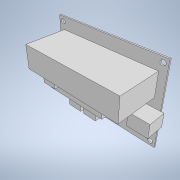
# Autodesk Inventor part: Плата
Saved by Autodesk Inventor 2021.1 (Build 251245010, 245A)
## iProperties
Created: 2026-06-02
Part Number: Плата
Material: Типовые
Document SubType Name: Modeling
Designer: Андрей Тарасов
Density: 1 g/cm^3
Appearance: По умолчанию
Author: Андрей Тарасов
Autodesk Inventor part; units mm, degrees
ref_plane "YZ Plane" through (0, 0, 0) normal (1, 0, 0) x (0, 1, 0)
ref_plane "XZ Plane" through (0, 0, 0) normal (0, 1, 0) x (-1, 0, 0)
ref_plane "XY Plane" through (0, 0, 0) normal (0, 0, 1) x (1, 0, 0)
sketch "Эскиз1" plane through (0, 0, 0) normal (0, 0, 1) x (1, 0, 0)
  line L0 (36.5, -27) -> (-36.5, -27)
  line L1 (-36.5, -27) -> (-36.5, 27)
  line L2 (-36.5, 27) -> (36.5, 27)
  line L3 (36.5, 27) -> (36.5, -27)
  line L4 (36.5, -27) -> (-36.5, 27) construction
  line L5 (-36.5, -27) -> (36.5, 27) construction
  circle A0 centre (-33.5, -24) radius 1.6
  circle A1 centre (-33.5, 24) radius 1.6
  circle A2 centre (33.5, 24) radius 1.6
  circle A3 centre (33.5, -24) radius 1.6
  line L6 (-35.1, 24) -> (36.5, 24) construction
  line L7 (-33.5, 27) -> (-33.5, -27) construction
  line L8 (-36.5, -24) -> (36.5, -24) construction
  line L9 (33.5, 27) -> (33.5, -27) construction
  point P0 (0, 0)
  dimension "d6" = 3.2
  dimension "d0" = 73
  dimension "d1" = 54
  dimension "d2" = 3
  dimension "d3" = 3
  dimension "d4" = 3
  dimension "d5" = 3
  constraints: 20 end point, 15 point on line, 5 perpendicular, 3 centre point, 2 equal radius, 2 midpoint, 2 parallel, 1 horizontal, 1 horizontal alignment, 3 other
  measures "d0" distance of L1.end L2.end
  measures "d1" distance of L0.end L1.end
  measures "d2" distance between parallel lines of L2 L6
  measures "d3" distance between parallel lines of L1 L7
  measures "d4" distance between parallel lines of L3 L9
  measures "d5" distance between parallel lines of L0 L8
extrude "Выдавливание1" add sketch "Эскиз1" along normal blind 1
sketch "Эскиз2" plane through (0, 0, 1) normal (0, 0, 1) x (1, 0, 0)
  line L0 (25.5, -2) -> (38.5, -2)
  line L1 (38.5, -2) -> (38.5, -11)
  line L2 (38.5, -11) -> (25.5, -11)
  line L3 (25.5, -11) -> (25.5, -2)
  line L4 (-36.5, -27) -> (36.5, -27) projected
  line L5 (36.5, -27) -> (36.5, 27) projected
  point P0 (0, 0)
  dimension "d9" = 13
  dimension "d10" = 9
  dimension "d11" = 16
  dimension "d12" = 2
  constraints: 8 end point, 2 parallel, 1 horizontal, 1 perpendicular
  measures "d9" distance of L1.end L2.end
  measures "d10" distance of L0.end L1.end
  measures "d11" distance between parallel lines of L4 L2
  measures "d12" distance between parallel lines of L1 L5
extrude "Выдавливание2" add sketch "Эскиз2" along normal blind 11.5
sketch "Эскиз3" plane through (0, 0, 1) normal (0, 0, 1) x (1, 0, 0)
  line L0 (-24.5, -28) -> (-1.5, -28)
  line L1 (-1.5, -28) -> (-1.5, -21)
  line L2 (-1.5, -21) -> (-24.5, -21)
  line L3 (-24.5, -21) -> (-24.5, -28)
  line L4 (-36.5, -27) -> (36.5, -27) projected
  line L5 (-36.5, 27) -> (-36.5, -27) projected
  line L6 (-14.25, -21) -> (-14.25, -28)
  line L7 (-11.75, -21) -> (-11.75, -28)
  point P0 (0, 0)
  dimension "d15" = 23
  dimension "d16" = 7
  dimension "d17" = 1
  dimension "d18" = 12
  dimension "d21" = 2.5
  dimension "d22" = 10.25
  constraints: 12 end point, 4 point on line, 3 perpendicular, 2 parallel, 1 horizontal
  measures "d15" distance of L1.end L2.end
  measures "d16" distance of L2.end L0.start
  measures "d17" distance between parallel lines of L0 L4
  measures "d18" distance between parallel lines of L5 L3
  measures "d21" distance between parallel lines of L7 L6
  measures "d22" distance between parallel lines of L6 L3
extrude "Выдавливание3" add sketch "Эскиз3" along normal blind 6 contours L3 L4 L6 L0 | L3 L2 L6 L4 | L7 L4 L1 L0 | L7 L2 L1 L4
sketch "Эскиз4" plane through (0, 0, 1) normal (0, 0, 1) x (1, 0, 0)
  line L0 (-33.5, 1) -> (9.5, 1)
  line L1 (9.5, 1) -> (9.5, -16)
  line L2 (9.5, -16) -> (-33.5, -16)
  line L3 (-33.5, -16) -> (-33.5, 1)
  line L4 (-36.5, -27) -> (-24.5, -27) projected
  line L5 (-36.5, 27) -> (-36.5, -27) projected
  point P0 (0, 0)
  dimension "d23" = 17
  dimension "d24" = 43
  dimension "d25" = 11
  dimension "d26" = 3
  constraints: 8 end point, 2 parallel, 1 horizontal, 1 perpendicular
  measures "d23" distance of L2.end L0.start
  measures "d24" distance of L0.start L0.end
  measures "d25" distance between parallel lines of L2 L4
  measures "d26" distance between parallel lines of L3 L5
extrude "Выдавливание4" add sketch "Эскиз4" along normal blind 12.5
sketch "Эскиз5" plane through (0, 0, 13.5) normal (0, 0, 1) x (1, 0, 0)
  line L0 (-25, -11) -> (-35, -11)
  line L1 (-35, -11) -> (-35, -4)
  line L2 (-35, -4) -> (-25, -4)
  line L3 (-25, -4) -> (-25, -11)
  line L4 (-25, -11) -> (-35, -4) construction
  line L5 (-35, -11) -> (-25, -4) construction
  line L6 (-35, -7.5) -> (-25, -7.5) construction
  line L7 (-33.5, 1) -> (-33.5, -16) projected
  point P0 (0, 0)
  point P1 (-30, -7.5)
  point P2 (-33.5, -7.5)
  dimension "d29" = 10
  dimension "d30" = 7
  dimension "d31" = 1.5
  constraints: 14 end point, 5 midpoint, 2 parallel, 1 horizontal, 1 perpendicular, 1 point on line
  measures "d29" distance of L1.end L2.end
  measures "d30" distance of L0.end L1.end
  measures "d31" distance between parallel lines of L7 L1
extrude "Выдавливание5" add sketch "Эскиз5" along normal blind 4
sketch "Эскиз6" plane through (0, 0, 1) normal (0, 0, 1) x (1, 0, 0)
  line L0 (32, 19) -> (-33, 19)
  line L1 (-33, 19) -> (-33, 4)
  line L2 (-33, 4) -> (32, 4)
  line L3 (32, 4) -> (32, 19)
  line L4 (36.5, 27) -> (-36.5, 27) projected
  line L5 (-36.5, 27) -> (-36.5, -27) projected
  point P0 (0, 0)
  dimension "d34" = 15
  dimension "d35" = 65
  dimension "d36" = 8
  dimension "d37" = 3.5
  constraints: 8 end point, 2 parallel, 1 horizontal, 1 perpendicular
  measures "d34" distance between parallel lines of L2 L0
  measures "d35" distance of L0.start L0.end
  measures "d36" distance between parallel lines of L0 L4
  measures "d37" distance between parallel lines of L5 L1
extrude "Выдавливание6" add sketch "Эскиз6" along normal blind 27
equation "\"d3\" = d2"
equation "\"d4\" = d2"
equation "\"d5\" = d2"
equation "\"d22\" = -0.5 * d21 + 0.5 * d15"
